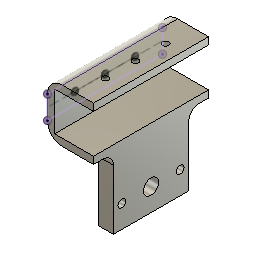
y leadscrewholder endstop (Autodesk Fusion 360 design; units mm, degrees)
Autodesk Fusion 360 part; units mm, degrees
sketch "Sketch1" plane through (0, 0, 0) normal (0, 0, 1) x (1, 0, 0)
  line L0 (0, 0) -> (25.8, 0)
  line L1 (25.8, 0) -> (25.8, -25.8)
  line L2 (0, 0) -> (25.8, 0)
  line L3 (25.8, 0) -> (25.8, -25.8)
  line L4 (25.8, -25.8) -> (0, -25.8)
  line L5 (0, -25.8) -> (0, 0)
  line L6 (25.8, -30.55) -> (-4.75, -30.55)
  line L7 (-4.75, -30.55) -> (-4.75, 4.75)
  line L8 (-4.75, 4.75) -> (25.8, 4.75)
  line L9 (25.8, 0) -> (25.8, 4.75)
  line L10 (25.8, 4.75) -> (25.8, -30.55)
  line L11 (25.8, -12.9) -> (25.8, -62.331)
  line L12 (25.8, -62.331) -> (25.8, -77.331)
  line L13 (25.8, -62.331) -> (25.8, -47.331)
  line L14 (25.8, -47.331) -> (15.8, -47.331)
  line L15 (15.8, -47.331) -> (15.8, -30.55)
  line L16 (15.8, -47.331) -> (15.8, -77.331)
  line L17 (25.8, -77.331) -> (15.8, -77.331)
  dimension "d1" = 25.8
  dimension "d2" = 25.8
  dimension "d4" = 49.431
  dimension "d5" = 15
  dimension "d6" = 15
  dimension "d7" = 10
  constraint coincident L0.start L2.start
  constraint horizontal L0
  constraint perpendicular L0 L1
  constraint horizontal L2
  constraint vertical L3
  constraint horizontal L4
  constraint vertical L5
  constraint perpendicular L8 L9
  constraint perpendicular L6 L10
  constraint midpoint L3 L11.start
  constraint perpendicular L6 L11
  constraint perpendicular L6 L12
  constraint parallel L11 L13
  constraint perpendicular L11 L14
  constraint coincident L6 L15.end
  constraint perpendicular L6 L15
  constraint perpendicular L6 L16
  constraint perpendicular L16 L17
  measures "d1" distance of L0.start L0.end
  measures "d2" distance of L0.end L1.end
  measures "d4" distance of L11.start L11.end
  measures "d5" distance of L11.end L12.end
  measures "d6" distance of L11.end L13.end
  measures "d7" distance of L13.end L14.end
extrude "Extrude1" add sketch "Sketch1" along normal blind 76.4 contours L0 L2 L4 L5 L6 L7 L8 L9 L10 L11
ref_plane "WorkPlane1" through (10.525, -12.9, 38.2) normal (0, 0, 1) x (1, 0, 0)
extrude "Extrude2" add sketch "Sketch1" along normal mid plane 50 from surface at 38.2 contours L6 L11 L14 L15 | L11 L12 L13 L14 L16 L17
sketch "Sketch2" plane through (15.8, 0, 0) normal (-1, 0, 0) x (0, 0, 1)
  line L0 (13.2, -77.331) -> (63.2, -77.331)
  line L1 (63.2, -77.331) -> (63.2, -30.55)
  line L2 (63.2, -30.55) -> (13.2, -30.55)
  line L3 (13.2, -30.55) -> (13.2, -77.331)
  line L4 (0, -47.331) -> (0, -77.331)
  line L5 (0, -62.331) -> (0, -77.331)
  line L6 (0, -62.331) -> (0, -47.331)
  line L7 (0, -77.331) -> (0, -62.331)
  line L8 (13.2, -62.331) -> (63.2, -62.331) construction
  circle A0 centre (38.2, -62.331) radius 5
  line L9 (63.2, -62.331) -> (60.2, -62.331)
  circle A1 centre (57.65, -62.331) radius 2.55
  line L10 (38.2, -62.331) -> (38.2, -60) construction
  circle A2 centre (18.75, -62.331) radius 2.55
  dimension "d13" = 10
  dimension "d14" = 3
  dimension "d15" = 5.1
  constraint coincident L4.end L5.end
  constraint coincident L5.start L6.start
  constraint coincident L1 L8.end
  constraint perpendicular L1 L8
  constraint coincident L3 L8.start
  constraint midpoint L8 A0.centre
  constraint perpendicular L1 L9
  constraint coincident L9.end A1
  constraint coincident A0.centre L10.start
  constraint perpendicular L8 L10
  constraint symmetric A1 L10 A2
  measures "d13" diameter of A0
  measures "d14" distance of L8.end L9.end
  measures "d15" diameter of A1
extrude "Extrude3" cut sketch "Sketch2" against normal blind 61 contours A0 | A1 | A2
fillet "Fillet1" radius 10 2 edges at (-4.75, -30.55, 38.2) (-4.75, 4.75, 38.2)
fillet "Fillet2" radius 7 2 edges at (20.8, -30.55, 63.2) (20.8, -30.55, 13.2)
fillet "Fillet3" radius 10.5 1 edges at (15.8, -30.55, 38.2)
sketch "Sketch3" plane through (-4.75, 0, 0) normal (-1, 0, 0) x (0, 0, 1)
  line L0 (76.4, -5.25) -> (0, -5.25)
  line L1 (0, -5.25) -> (0, -20.55)
  line L2 (0, -20.55) -> (76.4, -20.55)
  line L3 (76.4, -20.55) -> (76.4, -5.25)
  line L4 (0, -12.9) -> (76.4, -12.9) construction
  circle A0 centre (38.2, -12.9) radius 2.1
  line L5 (38.2, -12.9) -> (58.2, -12.9) construction
  circle A1 centre (58.2, -12.9) radius 2.1
  line L6 (38.2, -12.9) -> (18.2, -12.9) construction
  circle A2 centre (18.2, -12.9) radius 2.1
  dimension "d24" = 4.2
  dimension "d25" = 20
  dimension "d26" = 4.2
  dimension "d27" = 20
  dimension "d28" = 4.2
  constraint midpoint L1 L4.start
  constraint midpoint L3 L4.end
  constraint midpoint L4 A0.centre
  constraint coincident A0.centre L5.start
  constraint coincident L4 L5.end
  constraint coincident L5.end A1.centre
  constraint parallel L4 L6
  constraint coincident L6.end A2.centre
  measures "d24" diameter of A0
  measures "d25" distance of A0.centre L5.end
  measures "d26" diameter of A1
  measures "d27" distance of A0.centre L6.end
  measures "d28" diameter of A2
extrude "Extrude4" cut sketch "Sketch3" against normal blind 40 contours A0 | A1 | A2
sketch "Sketch4" plane through (0, 4.75, 0) normal (0, 1, 0) x (-1, 0, 0)
  line L0 (-5.25, 0) -> (-5.25, 76.4)
  line L1 (-5.25, 76.4) -> (-25.8, 76.4)
  line L2 (-25.8, 76.4) -> (-25.8, 0)
  line L3 (-25.8, 0) -> (-5.25, 0)
  line L4 (4.75, 36.1) -> (4.75, 40.3)
  line L5 (4.75, 16.1) -> (4.75, 20.3)
  line L6 (4.75, 56.1) -> (4.75, 60.3)
  line L7 (4.75, 18.2) -> (-25.8, 18.2) construction
  line L8 (4.75, 38.2) -> (-25.8, 38.2) construction
  line L9 (4.75, 58.2) -> (-25.8, 58.2) construction
  line L10 (-25.8, 18.2) -> (-5.25, 18.2) construction
  line L11 (-5.25, 38.2) -> (-25.8, 38.2)
  line L12 (-25.8, 58.2) -> (-5.25, 58.2)
  circle A0 centre (-15.525, 18.2) radius 2.1
  circle A1 centre (-15.525, 38.2) radius 2.1
  circle A2 centre (-15.525, 58.2) radius 2.1
  point P0 (4.75, 18.2)
  dimension "d31" = 4.2
  dimension "d32" = 4.2
  dimension "d33" = 4.2
  constraint coincident P0 L7.start
  constraint coincident L2 L7.end
  constraint perpendicular L2 L7
  constraint midpoint L4 L8.start
  constraint midpoint L2 L8.end
  constraint midpoint L6 L9.start
  constraint coincident L2 L9.end
  constraint perpendicular L2 L9
  constraint coincident L7 L10.end
  constraint coincident L0 L10.end
  constraint midpoint L0 L11.start
  constraint coincident L0 L12.end
  constraint coincident L9 L12.end
  constraint midpoint L10 A0.centre
  constraint midpoint L11 A1.centre
  constraint midpoint L12 A2.centre
  measures "d31" diameter of A0
  measures "d32" diameter of A1
  measures "d33" diameter of A2
extrude "Extrude5" cut sketch "Sketch4" against normal blind 15 contours L11 A1 | L11 A1 | L12 A2 | L12 A2 | A0
